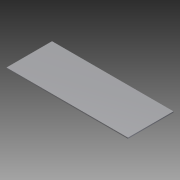
# Autodesk Inventor part: ElectronicsBoardVerticalBottom
Saved by Autodesk Inventor 2012 (Build 160160000, 160)
## iProperties
Created: 2012-01-10
Part Number: ElectronicsBoardVerticalBottom
Material: Default
Document SubType Name: Modeling
Designer: William
Density: 1 g/cm^3
Author: William
Autodesk Inventor part; units mm, degrees
ref_plane "YZ Plane" through (0, 0, 0) normal (1, 0, 0) x (0, 1, 0)
ref_plane "XZ Plane" through (0, 0, 0) normal (0, 1, 0) x (-1, 0, 0)
ref_plane "XY Plane" through (0, 0, 0) normal (0, 0, 1) x (1, 0, 0)
sketch "Sketch1" plane through (0, 0, 0) normal (0, 0, 1) x (1, 0, 0)
  line L0 (185.4498, -59.7201) -> (-424.1502, -59.7201)
  line L1 (-424.1502, -59.7201) -> (-424.1502, -54.6401)
  line L2 (-424.1502, -54.6401) -> (185.4498, -54.6401)
  line L3 (185.4498, -54.6401) -> (185.4498, -59.7201)
  point P0 (0, 0)
  dimension "d0" = 609.6
  dimension "d1" = 5.08
  constraints: 8 end point, 2 parallel, 1 horizontal, 1 perpendicular
  measures "d0" distance of L1.end L2.end
  measures "d1" distance of L0.end L1.end
extrude "Extrusion1" add sketch "Sketch1" along normal blind 228.6
body "Solid1"
